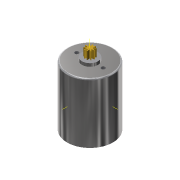
# Autodesk Inventor part: empty
Saved by Autodesk Inventor 2014 (Build 180170000, 170)
## iProperties
Created: 2015-04-13
Part Number: empty
Material: Generic
Document SubType Name: Modeling
Designer: Martin
Density: 1 g/cm^3
Appearance: Default
Author: Martin
Autodesk Inventor part; units mm, degrees
ref_plane "YZ Plane" through (0, 0, 0) normal (1, 0, 0) x (0, 1, 0)
ref_plane "XZ Plane" through (0, 0, 0) normal (0, 1, 0) x (-1, 0, 0)
ref_plane "XY Plane" through (0, 0, 0) normal (0, 0, 1) x (1, 0, 0)
sketch "Sketch1" plane through (0, 0, 0) normal (0, 1, 0) x (-1, 0, 0)
  line L0 (0, -22.2029) -> (0, 22.4648) projected
  line L1 (10.56, 0) -> (-1.76, 0) projected
  line L2 (0, 16.0837) -> (0, -15.8218)
  line L3 (0, -11.9411) -> (8.8, -11.9411)
  line L4 (8.8, -11.9411) -> (8.8, 11.0589)
  line L5 (8.8, 11.0589) -> (3.075, 11.0589)
  line L6 (3.075, 11.0589) -> (3.075, 12.2589)
  line L7 (3.075, 12.2589) -> (1.825, 12.2589)
  line L8 (1.825, 12.2589) -> (1.825, 15.2589)
  line L9 (1.825, 15.2589) -> (0, 15.2589)
  line L10 (0, -11.9411) -> (0, 15.2589)
  line L11 (0, -12.9411) -> (2.35, -12.9411)
  line L12 (2.35, -12.9411) -> (2.35, -11.9411)
  line L13 (0, -11.9411) -> (0, -12.9411)
  point P0 (0, 0)
  dimension "d0" = 17.6
  dimension "d1" = 23
  dimension "d2" = 1
  dimension "d3" = 4.7
  dimension "d4" = 6.15
  dimension "d5" = 3.65
  dimension "d6" = 1.2
  dimension "d7" = 3
  constraints: 24 end point, 6 point on line, 5 perpendicular, 4 parallel, 2 collinear
  measures "d0" diameter of L4 L2
  measures "d1" distance of L3.end L4.end
  measures "d2" distance of L11.end L12.end
  measures "d3" diameter of L12 L2
  measures "d4" diameter of L6 L2
  measures "d5" diameter of L8 L2
  measures "d6" distance of L5.end L6.end
  measures "d7" distance of L7.end L8.end
revolve "Revolution1" add sketch "Sketch1" angle 360 about axis through (0, 0, -10) along (0, 0, 1)
sketch "Sketch2" plane through (0, 0, 11.0589) normal (0, 0, 1) x (1, 0, 0)
  line L0 (-12.32, 0) -> (12.32, 0) projected
  circle A0 centre (-5.075, 0) radius 0.725
  circle A1 centre (5.075, 0) radius 0.725
  line L1 (0, -12.32) -> (0, 12.32) projected
  dimension "d9" = 1.45
  dimension "d10" = 10.15
  constraints: 2 centre point, 2 point on line, 1 equal radius, 1 symmetric about line
  measures "d9" diameter of A0
  measures "d10" distance of A1.centre A0.centre
extrude "Extrusion1" cut sketch "Sketch2" against normal blind 10
sketch "Sketch3" plane through (0, 0, -11.9411) normal (0, 0, -1) x (-1, 0, 0)
  line L0 (12.32, 0) -> (-12.32, 0) projected
  line L1 (0, -12.32) -> (0, 12.32) projected
  line L2 (-2, 7) -> (2, 7)
  line L3 (2, 7) -> (2, 5)
  line L4 (2, 5) -> (-2, 5)
  line L5 (-2, 5) -> (-2, 7)
  line L6 (-2, 7) -> (2, 5) construction
  line L7 (2, 7) -> (-2, 5) construction
  line L8 (-2, -7) -> (2, -7)
  line L9 (2, -7) -> (2, -5)
  line L10 (2, -5) -> (-2, -5)
  line L11 (-2, -5) -> (-2, -7)
  line L12 (-2, -7) -> (2, -5) construction
  line L13 (2, -7) -> (-2, -5) construction
  point P0 (0, 6)
  point P1 (0, -6)
  dimension "d13" = 4
  dimension "d14" = 14
  dimension "d15" = 2
  constraints: 24 end point, 4 midpoint, 4 parallel, 2 horizontal, 2 perpendicular, 2 point on line, 4 other
  measures "d13" distance of L2.start L2.end
  measures "d14" distance between parallel lines of L8 L2
  measures "d15" distance of L2.end L3.end
extrude "Extrusion2" add sketch "Sketch3" along normal blind 1
sketch "Sketch4" plane through (0, 0, 15.2589) normal (0, 0, 1) x (1, 0, 0)
  circle A0 centre (0, 0) radius 1.825 projected
  line L0 (0, -12.32) -> (0, 12.32) projected
  line L1 (-12.32, 0) -> (12.32, 0) projected
  line L2 (-0.4802, 1.7607) -> (0, 0.7709)
  line L3 (0.4802, 1.7607) -> (0, 0.7709)
  line L4 (0, 0) -> (-0.564, 1.7357) construction
  line L5 (0, 0) -> (0.564, 1.7357) construction
  arc A1 (-0.09, 0.9564) -> (0.09, 0.9564) centre (0, 1) ccw
  arc A2 (-0.4431, 1.6842) -> (-0.564, 1.7357) centre (-0.5331, 1.6406) ccw
  arc A3 (0.564, 1.7357) -> (0.4431, 1.6842) centre (0.5331, 1.6406) ccw
  line L6 (0, 1) -> (0, 1.825)
  dimension "d18" = 0.1
  dimension "d19" = 36
  dimension "d22" = 0.1
  dimension "d29" = 0.825
  constraints: 11 point on circle, 10 end point, 6 point on line, 3 centre point, 3 tangent, 1 line through centre, 3 other
  measures "d18" radius of A1
  measures "d19" angle of L5 L4
  measures "d22" radius of A2
  measures "d29" distance of L6.start L6.end
extrude "Extrusion3" cut sketch "Sketch4" against normal up to surface (3 mm away) contours A3 L3 A0 | L3 A1 L0 A0 | L0 A1 L2 A0 | A0 L2 A2
pattern_circular "Circular Pattern1" count 10 over 360 about axis through (0, 0, -10) along (0, 0, 1) of "Extrusion3"
fillet "Fillet1" radius 0.5 1 edges at (8.8, 0, 11.0589)
body "Solid1"
